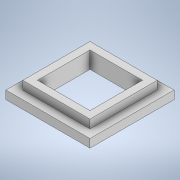
# Autodesk Inventor part: latticeChambercapv4
Saved by Autodesk Inventor 2020 (Build 240168000, 168)
## iProperties
Created: 2022-09-01
Part Number: latticeChambercapv4
Material: Generic
Document SubType Name: Modeling
Designer: ISS
Density: 1 g/cm^3
Appearance: Default
Author: ISS
Autodesk Inventor part; units mm, degrees
ref_plane "YZ Plane" through (0, 0, 0) normal (1, 0, 0) x (0, 1, 0)
ref_plane "XZ Plane" through (0, 0, 0) normal (0, 1, 0) x (-1, 0, 0)
ref_plane "XY Plane" through (0, 0, 0) normal (0, 0, 1) x (1, 0, 0)
sketch "Sketch10" plane through (0, 0, 0) normal (0, 1, 0) x (-1, 0, 0)
  line L0 (-11.8893, 0) -> (-31.8893, 0)
  line L1 (-31.8893, 0) -> (-31.8893, -20)
  line L2 (-31.8893, -20) -> (-11.8893, -20)
  line L3 (-11.8893, -20) -> (-11.8893, 0)
  line L4 (-11.8893, -20) -> (-31.8893, 0)
  line L5 (-31.8893, -20) -> (-11.8893, 0)
  line L6 (-21.8893, -10) -> (-28.1393, -10)
  line L7 (-28.1393, -10) -> (-28.1393, -16.25)
  line L8 (-28.1393, -16.25) -> (-21.8893, -16.25)
  line L9 (-21.8893, -16.25) -> (-21.8893, -10)
  line L10 (-28.1393, -16.25) -> (-15.6393, -16.25)
  line L11 (-15.6393, -16.25) -> (-15.6393, -3.75)
  line L12 (-15.6393, -3.75) -> (-28.1393, -3.75)
  line L13 (-28.1393, -3.75) -> (-28.1393, -16.25)
  point P0 (0, 0)
  dimension "d40" = 20
  dimension "d41" = 20
  dimension "d42" = 6.25
  dimension "d43" = 6.25
  dimension "d44" = 12.5
  dimension "d45" = 12.5
  constraints: 28 end point, 6 parallel, 3 horizontal, 3 perpendicular, 1 midpoint
  measures "d40" distance of L2.end L1.end
  measures "d41" distance of L1.end L0.end
  measures "d42" distance of L8.end L7.end
  measures "d43" distance of L7.end L6.end
  measures "d44" distance of L12.end L11.end
  measures "d45" distance of L11.end L10.end
extrude "Extrusion9" add sketch "Sketch10" along normal blind 2 contours L5 L12 L4 L0 | L3 L4 L11 L5 | L4 L13 L7 L5 L1 | L2 L5 L8 L10 L4
sketch "Sketch11" plane through (0, 2, 0) normal (0, 1, 0) x (1, 0, 0)
  line L0 (11.8893, 0) -> (31.8893, 0) projected
  line L1 (31.8893, 0) -> (31.8893, 20) projected
  line L2 (31.8893, 20) -> (11.8893, 20) projected
  line L3 (11.8893, 20) -> (11.8893, 0) projected
  line L4 (28.1393, 16.25) -> (28.1393, 3.75) projected
  line L5 (28.1393, 3.75) -> (15.6393, 3.75) projected
  line L6 (15.6393, 3.75) -> (15.6393, 16.25) projected
  line L7 (15.6393, 16.25) -> (28.1393, 16.25) projected
  line L8 (13.8893, 18) -> (29.8893, 18)
  line L9 (29.8893, 18) -> (29.8893, 2)
  line L10 (29.8893, 2) -> (13.8893, 2)
  line L11 (13.8893, 2) -> (13.8893, 18)
  point P0 (0, 0)
  dimension "d48" = 2
  constraints: 8 end point, 3 other
  measures "d48" distance between parallel lines of L2 L8
extrude "Extrusion10" add sketch "Sketch11" along normal blind 2 contours L8 L9 L10 L11
body "Solid1"
